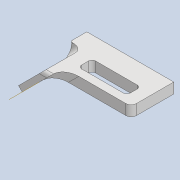
# Autodesk Inventor part: mot_holder_2
Saved by Autodesk Inventor 2020 (Build 240168000, 168)
## iProperties
Created: 2021-08-06
Part Number: mot_holder_2
Material: Generic
Document SubType Name: Modeling
Designer: Shuang Peng
Density: 1 g/cm^3
Appearance: Default
Author: Shuang Peng
Autodesk Inventor part; units mm, degrees
ref_plane "YZ Plane" through (0, 0, 0) normal (1, 0, 0) x (0, 1, 0)
ref_plane "XZ Plane" through (0, 0, 0) normal (0, 1, 0) x (-1, 0, 0)
ref_plane "XY Plane" through (0, 0, 0) normal (0, 0, 1) x (1, 0, 0)
sketch "Sketch1" plane through (0, 0, 0) normal (0, 0, 1) x (1, 0, 0)
  circle A0 centre (10, 45.25) radius 1 projected
  circle A1 centre (-10, 45.25) radius 1 projected
  circle A2 centre (20, 45.25) radius 1 projected
  circle A3 centre (-20, 45.25) radius 1 projected
  arc A4 (-11.1676, 34.8322) -> (-15.9868, 32.0083) centre (0, 10.25) ccw projected
  line L0 (-11.1676, 34.8322) -> (-14.1239, 40.0058) projected
  arc A5 (-12.8216, 42.25) -> (-14.1239, 40.0058) centre (-12.8216, 40.75) ccw projected
  line L1 (-12.8216, 42.25) -> (12.8216, 42.25) projected
  arc A6 (14.1239, 40.0058) -> (12.8216, 42.25) centre (12.8216, 40.75) ccw projected
  line L2 (14.1239, 40.0058) -> (11.1676, 34.8322) projected
  arc A7 (15.9868, 32.0083) -> (11.1676, 34.8322) centre (0, 10.25) ccw projected
  arc A8 (16.5122, 34.1074) -> (15.9868, 32.0083) centre (19.9851, 32.1228) ccw projected
  line L3 (16.5122, 34.1074) -> (20.0134, 40.2346) projected
  arc A9 (23.4864, 42.25) -> (20.0134, 40.2346) centre (23.4864, 38.25) ccw projected
  line L4 (23.4864, 42.25) -> (25, 42.25) projected
  line L5 (25, 42.25) -> (25, 48.25) projected
  line L6 (25, 48.25) -> (-25, 48.25) projected
  line L7 (-25, 48.25) -> (-25, 42.25) projected
  line L8 (-25, 42.25) -> (-23.4864, 42.25) projected
  arc A10 (-20.0134, 40.2346) -> (-23.4864, 42.25) centre (-23.4864, 38.25) ccw projected
  line L9 (-20.0134, 40.2346) -> (-16.5122, 34.1074) projected
  arc A11 (-15.9868, 32.0083) -> (-16.5122, 34.1074) centre (-19.9851, 32.1228) ccw projected
  line L10 (25, 48.25) -> (-25, 48.25)
  line L11 (-25, 48.25) -> (-25, 42.25)
  line L12 (-25, 42.25) -> (25, 42.25)
  line L13 (25, 42.25) -> (25, 48.25)
  point P0 (0, 0)
  point P1 (12.8216, 42.25)
  constraints: 8 end point, 2 parallel, 1 horizontal, 1 perpendicular
ref_plane "Work Plane1" through (-29.6985, 30.049, 24.5) normal (0, 0, -1) x (0, 1, 0)
extrude "Extrusion1" add sketch "Sketch1" along normal up to surface (24.5 mm away) contours L12 L8 L7 L6 L5 L4 L1
sketch "Sketch2" plane through (-25, 42.25, 24.5) normal (0, 0, 1) x (1, 0, 0)
  line L0 (0, 6) -> (0, 0) projected
  line L1 (0, 0) -> (50, 0) projected
  line L2 (50, 0) -> (50, 6) projected
  line L3 (50, 6) -> (0, 6) projected
  circle A0 centre (5, 3) radius 1 projected
  circle A1 centre (45, 3) radius 1 projected
  circle A2 centre (15, 3) radius 1 projected
  circle A3 centre (35, 3) radius 1 projected
  point P0 (25, -42.25)
extrude "Extrusion2" add sketch "Sketch2" against normal blind 18 contours A0 | A1 | A2 | A3
ref_plane "Work Plane2" through (-31.1127, 30.7561, 37.5) normal (-0.7071068, 0.7071068, 0) x (-0.7071068, -0.7071068, 0)
sketch "Sketch3" plane through (-31.1127, 30.7561, 37.5) normal (-0.7071068, 0.7071068, 0) x (-0.7071068, -0.7071068, 0)
  line L0 (0, -11) -> (-2, -13) projected
  line L1 (0, -4) -> (0, -11) projected
  line L2 (0, 0) -> (0, -4) projected
  line L3 (-15, 0) -> (0, 0) projected
  line L4 (-15, 0) -> (-15, -4) projected
  line L5 (-15, -4) -> (-15, -11) projected
  line L6 (-13, -13) -> (-15, -11) projected
  line L7 (-2, -13) -> (-13, -13) projected
  circle A0 centre (-3.5, -8.5) radius 1.6 projected
  circle A1 centre (-11.5, -8.5) radius 1.6 projected
  circle A2 centre (-11.5, -8.5) radius 1
  circle A3 centre (-3.5, -8.5) radius 1
  line L8 (0, 0) -> (0, -5)
  line L9 (0, -5) -> (-20, -5)
  line L10 (-20, -5) -> (-20, -13)
  line L11 (-20, -13) -> (0, -13)
  line L12 (0, -13) -> (0, -5)
  point P0 (-0.2522, -37.5)
  point P1 (-13, -13)
  point P2 (-2, -13)
  dimension "d4" = 2
  dimension "d5" = 2
  dimension "d6" = 5
  dimension "d7" = 20
  dimension "d8" = 8
  constraints: 10 end point, 2 centre point, 2 coincident, 2 parallel, 1 horizontal, 1 perpendicular, 1 point on line
  measures "d4" diameter of A2
  measures "d5" diameter of A3
  measures "d6" distance of L2.start L8.end
  measures "d7" distance of L11.end L10.end
  measures "d8" distance of L10.end L9.end
extrude "Extrusion3" add sketch "Sketch3" along normal blind 3 contours L12 L11 L0 | L0 L7 L6 L5 L9 L1 | L11 L10 L9 L5 L6 | A0 | A1
sketch "Sketch4" plane through (-31.1127, 30.7561, 32.5) normal (0, 0, 1) x (0.7071068, -0.7071068, 0)
  line L0 (0, 20) -> (0, 16.2548) projected
  line L1 (0, 16.2548) -> (31.5503, 47.8051) projected
  line L2 (31.5503, 47.8051) -> (27.3076, 52.0477) projected
  line L3 (27.3076, 52.0477) -> (-8.0477, 16.6924) projected
  line L4 (-8.0477, 16.6924) -> (-3.8051, 12.4497) projected
  line L5 (-3.8051, 12.4497) -> (-3, 13.2548) projected
  line L6 (-3, 13.2548) -> (-3, 20) projected
  line L7 (-3, 20) -> (0, 20) projected
  line L8 (-3, 20) -> (-3, 21.7401)
  line L9 (0, 20) -> (0, 16.2548) projected
  line L10 (0, 20) -> (0, 24.7401)
  line L11 (27.3076, 52.0477) -> (-8.0477, 16.6924) projected
  line L12 (-3, 0) -> (-3, 20) projected
  point P0 (43.7478, 0.2522)
  point P1 (0, 24.7401)
  constraints: 4 end point, 2 collinear, 2 point on line
extrude "Extrusion4" add sketch "Sketch4" against normal up to surface (8 mm away) contours L7 L8 L3 L10
sketch "Sketch5" plane through (-25, 42.25, 24.5) normal (0, 0, 1) x (1, 0, 0)
  line L0 (1.1386, 0) -> (7.1386, 6) projected
  line L1 (7.1386, 6) -> (0, 6) projected
  line L2 (0, 6) -> (0, 0) projected
  line L3 (0, 0) -> (1.1386, 0) projected
  point P0 (25, -42.25)
extrude "Extrusion5" cut sketch "Sketch5" against normal blind 15
sketch "Sketch6" plane through (-25, 48.25, 0) normal (0, 1, 0) x (1, 0, 0)
  line L0 (9, -16) -> (41, -16) projected
  line L1 (0, -9.5) -> (7.1386, -9.5) projected
  line L2 (7.1386, -9.5) -> (7.1386, -32.5) projected
  line L3 (11.3812, -32.5) -> (7.1386, -32.5) projected
  line L4 (11.3812, -32.5) -> (11.3812, -24.5) projected
  line L5 (50, -24.5) -> (11.3812, -24.5) projected
  line L6 (50, 0) -> (50, -24.5) projected
  line L7 (50, 0) -> (0, 0) projected
  line L8 (0, 0) -> (0, -9.5) projected
  line L9 (15, -20) -> (35, -20)
  line L10 (35, -20) -> (35, -12)
  line L11 (35, -12) -> (15, -12)
  line L12 (15, -12) -> (15, -20)
  line L13 (15, -20) -> (35, -12) construction
  line L14 (35, -20) -> (15, -12) construction
  point P0 (25, 0)
  point P1 (25, -16)
  dimension "d15" = 20
  dimension "d16" = 8
  constraints: 12 end point, 3 midpoint, 3 parallel, 1 perpendicular
  measures "d15" distance of L9.start L9.end
  measures "d16" distance of L10.end L9.end
extrude "Extrusion6" cut sketch "Sketch6" against normal blind 15 contours L12 L11 L10 L0 | L0 L10 L9 L12
fillet "Fillet1" radius 2 4 edges at (10, 45.25, 20) (-10, 45.25, 20) (-10, 45.25, 12) (10, 45.25, 12)
fillet "Fillet2" radius 6 1 edges at (-16.6188, 45.25, 24.5)
fillet "Fillet3" radius 2 1 edges at (-15.7401, 48.25, 32.5)
fillet "Fillet4" radius 4 1 edges at (-20.8614, 45.25, 9.5)
fillet "Fillet5" radius 1 2 edges at (-25, 47.5091, 9.5) (-25, 44.2438, 9.9204)
fillet "Fillet6" radius 3 1 edges at (-21.7401, 42.25, 24.5)
fillet "Fillet7" radius 3 2 edges at (-19.6188, 42.25, 23) (-19.6188, 42.25, 27.5)
chamfer "Chamfer1" distance 2 angle 45 2 edges at (-32.1734, 31.8168, 32.5) (-32.1734, 31.8168, 24.5)
thicken "Thicken1" operation add thickness 8 both sides no extend neighbours yes toward (1, 0, 0) faces at (10, 46.25, 16.6667)
fillet "Fillet8" radius 3 1 edges at (25, 45.25, 24.5)
body "Solid1"
